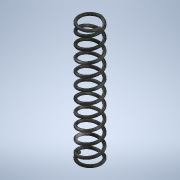
# Autodesk Inventor part: Spring 2
Saved by Autodesk Inventor 2020.1 (Build 241239000, 239)
## iProperties
Created: 2019-08-16
Part Number: Spring 2
Material: Steel
Document SubType Name: Modeling
Designer: Petar
Density: 7.85 g/cm^3
Appearance: Plate
Author: Petar
Autodesk Inventor part; units mm, degrees
ref_plane "YZ Plane" through (0, 0, 0) normal (1, 0, 0) x (0, 1, 0)
ref_plane "XZ Plane" through (0, 0, 0) normal (0, 1, 0) x (-1, 0, 0)
ref_plane "XY Plane" through (0, 0, 0) normal (0, 0, 1) x (1, 0, 0)
sketch "Sketch1" plane through (0, 0, 0) normal (1, 0, 0) x (0, 1, 0)
  line L0 (0, 0) -> (13.88, 0) construction
  circle A0 centre (13.72, -1.2) radius 0.16
  line L1 (13.88, 0) -> (13.88, -1.2) construction
  dimension "d1" = 0.32
  dimension "d0" = 13.88
  dimension "d2" = 1.2
  constraints: 4 end point, 1 horizontal, 1 horizontal alignment, 1 perpendicular, 1 vertical, 2 other
  measures "d0" distance of L0.start L0.end
  measures "d2" distance from line of L0 point (13.72, -1.2)
coil "Coil1" sketch "Sketch1" operation add axis through (0, 0, 0) along (0, -1, 0) pitch 1.356 turns 10 hand right
sketch "Sketch2" plane through (0, 13.72, -1.2) normal (-1, 0, 0) x (0, 0, 1)
  circle A0 centre (0, 0) radius 0.16 projected
  line L0 (1.2, -13.72) -> (1.2, 0.16) construction
  point P0 (0, 0.16)
  constraints: 1 vertical alignment
revolve "Revolution1" add sketch "Sketch2" angle 270 about axis through (0, 0, 0) along (0, 1, 0)
sketch "Sketch3" plane through (0, 0.16, -1.2) normal (1, 0, 0) x (0, 0, -1)
  circle A0 centre (0, 0) radius 0.16 projected
  line L0 (-1.2, -0.16) -> (-1.2, 13.72) construction
  point P0 (0, 0.16)
  constraints: 1 vertical alignment
revolve "Revolution2" add sketch "Sketch3" angle 270 about axis through (0, 0, 0) along (0, -1, 0)
equation "\"d3\" = -0.1 * d1 + 0.1 * d0"
body "Solid1"
